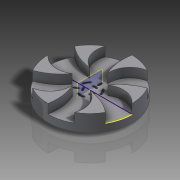
# Autodesk Inventor part: Impeller
Saved by Autodesk Inventor 2018.2 (Build 222227000, 227)
## iProperties
Created: 2018-02-02
Part Number: Impeller
Material: Generic
Document SubType Name: Modeling
Designer: Rus
Density: 1 g/cm^3
Appearance: Default
Author: Rus
Autodesk Inventor part; units mm, degrees
ref_plane "YZ Plane" through (0, 0, 0) normal (1, 0, 0) x (0, 1, 0)
ref_plane "XZ Plane" through (0, 0, 0) normal (0, 1, 0) x (-1, 0, 0)
ref_plane "XY Plane" through (0, 0, 0) normal (0, 0, 1) x (1, 0, 0)
sketch "Sketch1" plane through (0, 0, 0) normal (0, 1, 0) x (-1, 0, 0)
  circle A0 centre (0, 0) radius 38.1
  dimension "d0" = 76.2
  constraints: 1 centre point, 1 coincident
  measures "d0" diameter of A0
extrude "Extrusion1" add sketch "Sketch1" along normal blind 5.08 and the other way blind 1.5875
sketch "Sketch2" plane through (0, 5.08, 0) normal (0, 1, 0) x (1, 0, 0)
  circle A0 centre (0, 0) radius 38.1 construction
  circle A1 centre (0, 0) radius 38.1 construction
  line L0 (0, 0) -> (0, -38.1) construction
  arc A2 (-19.05, -32.9956) -> (0, -38.1) centre (0, 0) ccw
  arc A3 (-19.05, -32.9956) -> (-3.175, -12.7) centre (-22.2717, -14.1191) ccw
  arc A4 (0, -38.1) -> (-3.175, -12.7) centre (-42.8055, -30.5522) ccw
  line L1 (-3.175, -12.7) -> (-8.0548, -1.8672) construction
  line L2 (-3.175, -12.7) -> (-3.5133, -8.1478) construction
  line L3 (0, -38.1) -> (-0.6729, -41.9165) construction
  dimension "d22" = 30
  dimension "d27" = 3.175
  dimension "d28" = 12.7
  dimension "d29" = 20
  dimension "d30" = 10
  constraints: 8 end point, 8 point on circle, 3 centre point, 3 tangent, 1 coincident, 1 concentric, 1 vertical
  measures "d27" horizontal distance of point (0, 0) L1.start
  measures "d28" vertical distance of L1.start point (0, 0)
  measures "d29" angle of L1 L2
  measures "d30" angle of L3 L0
extrude "Extrusion2" add sketch "Sketch2" along normal blind 8.4667
pattern_circular "Circular Pattern3" count 6 over 360 about axis through (0, 0, 0) along (0, 1, 0) of "Extrusion2"
sketch "Sketch5" plane through (0, -1.5875, 0) normal (0, -1, 0) x (1, 0, 0)
  line L0 (-9.525, -5.4993) -> (0, 10.9985) construction
  line L1 (0, 10.9985) -> (9.525, -5.4993) construction
  line L2 (9.525, -5.4993) -> (-9.525, -5.4993) construction
  line L3 (0, 0) -> (0, 10.9985) construction
  arc A0 (-7.1044, 19.4652) -> (5.4993, 7.8235) centre (15.1901, 30.9585) ccw construction
  arc A1 (-9.9264, 18.0104) -> (4.2726, 4.8951) centre (15.1901, 30.9585) ccw
  arc A2 (-4.2823, 20.92) -> (6.7259, 10.752) centre (15.1901, 30.9585) ccw
  arc A3 (-4.2823, 20.92) -> (-9.9264, 18.0104) centre (-7.1044, 19.4652) ccw
  arc A4 (4.2726, 4.8951) -> (6.7259, 10.752) centre (5.4993, 7.8235) ccw
  arc A5 (-7.1044, 19.4652) -> (5.4993, 7.8235) centre (15.1901, 30.9585) ccw construction
  arc A6 (-8.2332, 18.8833) -> (5.0086, 6.6521) centre (15.1901, 30.9585) ccw
  arc A7 (-5.9755, 20.0471) -> (5.9899, 8.9949) centre (15.1901, 30.9585) ccw
  arc A8 (-5.9755, 20.0471) -> (-8.2332, 18.8833) centre (-7.1044, 19.4652) ccw
  arc A9 (5.0086, 6.6521) -> (5.9899, 8.9949) centre (5.4993, 7.8235) ccw
  dimension "d41" = 19.05
  dimension "d45" = 6.35
  dimension "d46" = 30
  dimension "d47" = 110
  dimension "d48" = 2.54
  dimension "d49" = 3.175
  dimension "d50" = 8.4667
  constraints: 22 point on circle, 10 centre point, 8 end point, 8 tangent, 2 coincident, 2 concentric, 1 horizontal, 1 vertical, 7 other
  measures "d41" distance of L1.end L0.start
  measures "d45" radial gap between concentric circles of A2 A1
  measures "d48" diameter of A9
  measures "d49" vertical distance of L0.end A0.end
  measures "d50" vertical distance of L0.end A0.start
extrude "Extrusion3" cut sketch "Sketch5" against normal blind 2.2225
pattern_circular "Circular Pattern4" count 3 over 360 about axis through (0, 0, 0) along (0, 1, 0) of "Extrusion3"
sketch "Sketch8" plane through (0, 5.08, 0) normal (0, 1, 0) x (1, 0, 0)
  arc A0 (32.9956, -19.05) -> (38.1, 0) centre (0, 0) ccw projected
  line L0 (38.1, 0) -> (-38.1, 0)
  constraints: 2 end point, 1 horizontal
ref_plane "Work Plane1" through (0, 5.08, 0) normal (-1, 0, 0) x (0, -1, 0)
sketch "Sketch9" plane through (0, 5.08, 0) normal (0, 1, 0) x (1, 0, 0)
  arc A0 (-2.546, -8.0748) -> (2.546, -8.0748) centre (0, 0) ccw construction
  arc A1 (-2.8006, -8.8823) -> (2.8006, -8.8823) centre (0, 0) ccw
  arc A2 (-2.2914, -7.2673) -> (2.2914, -7.2673) centre (0, 0) ccw
  arc A3 (-2.2914, -7.2673) -> (-2.8006, -8.8823) centre (-2.546, -8.0748) ccw
  arc A4 (2.8006, -8.8823) -> (2.2914, -7.2673) centre (2.546, -8.0748) ccw
  line L0 (0, 0) -> (-2.546, -8.0748) construction
  line L1 (0, 0) -> (2.546, -8.0748) construction
  arc A5 (1.1665, 3.6998) -> (1.6757, 5.3148) centre (1.4211, 4.5073) ccw
  arc A6 (1.6757, 5.3148) -> (-1.6757, 5.3148) centre (0, 0) ccw
  arc A7 (-1.6757, 5.3148) -> (-1.1665, 3.6998) centre (-1.4211, 4.5073) ccw
  arc A8 (1.1665, 3.6998) -> (-1.1665, 3.6998) centre (0, 0) ccw
  arc A9 (0.8467, 10.6106) -> (-0.8467, 10.6106) centre (0, 10.6106) ccw
  line L2 (-0.8467, 10.6106) -> (-0.8467, 7.6894)
  arc A10 (-0.8467, 7.6894) -> (0.8467, 7.6894) centre (0, 7.6894) ccw
  line L3 (0.8467, 7.6894) -> (0.8467, 10.6106)
  circle A11 centre (0, 0) radius 12.7273
  line L4 (-1.4211, 4.5073) -> (1.4211, 4.5073) construction
  point P0 (0, -8.4667)
  point P1 (0, 4.5073)
  dimension "d55" = 35
  dimension "d57" = 8.4667
  dimension "d58" = 0.8467
  dimension "d59" = 35
  dimension "d60" = 0.8467
  dimension "d61" = 4.726
  dimension "d62" = 25.4546
  dimension "d63" = 1.27
  dimension "d64" = 1.6933
  dimension "d65" = 0.8467
  dimension "d66" = 1.27
  dimension "d67" = 1.6933
  constraints: 23 point on circle, 12 centre point, 10 end point, 8 tangent, 4 vertical alignment, 2 coincident, 2 equal radius, 1 concentric, 1 horizontal, 1 midpoint, 1 parallel
  measures "d55" angle of L0 L1
  measures "d57" distance of point (0, -8.467) point (0, 0)
  measures "d58" radius of A4
  measures "d60" radius of A5
  measures "d61" distance of point (0, 0) L4.end
  measures "d62" diameter of A11
  measures "d64" distance between parallel lines of L2 L3
  measures "d65" radius of A9
  measures "d67" radial gap between concentric circles of A6 A8
extrude "Extrusion5" cut sketch "Sketch9" against normal blind 2 contours A3 A2 A4 A1 | A8 A7 A6 A5 | L3 A10 L2 A9
pattern_circular "Circular Pattern5" count 3 over 360 about axis through (0, 0, 0) along (0, 1, 0) of "Extrusion5"
body "Solid1"
